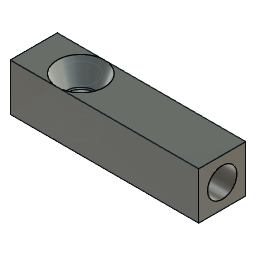
support_tige_metal (Autodesk Fusion 360 design; units mm, degrees)
Autodesk Fusion 360 part; units mm, degrees
sketch "Esquisse1" plane through (0, 0, 0) normal (0, 0, 1) x (1, 0, 0)
  line L0 (0, 0) -> (40, 0)
  line L1 (40, 0) -> (40, -10)
  line L2 (40, -10) -> (0, -10)
  line L3 (0, -10) -> (0, 0)
  circle A0 centre (10, -5) radius 3.25
  dimension "d1" = 6.5
  constraint horizontal L0
  constraint vertical L1
  constraint horizontal L2
  constraint vertical L3
  constraint coincident L0.start L3.end
  measures "d1" diameter of A0
extrude "Extrusion1" add sketch "Esquisse1" along normal blind 10
sketch "Esquisse2" plane through (40, 0, 0) normal (1, 0, 0) x (0, 1, 0)
  line L0 (-10, 0) -> (0, 0)
  line L1 (0, 0) -> (0, 10)
  line L2 (0, 10) -> (-10, 10)
  line L3 (-10, 10) -> (-10, 0)
  circle A0 centre (-5, 5) radius 3.1
  dimension "d4" = 6.2
  measures "d4" diameter of A0
extrude "Extrusion2" cut sketch "Esquisse2" against normal blind 20 contours A0
sketch "Esquisse3" plane through (0, 0, 10) normal (0, 0, 1) x (-1, 0, 0)
  circle A0 centre (-10, 5) radius 3.25
  line L0 (0, 10) -> (-40, 10)
  line L1 (-40, 10) -> (-40, 0)
  line L2 (-40, 0) -> (0, 0)
  line L3 (0, 0) -> (0, 10)
sketch "Esquisse4" plane through (0, 0, 0) normal (0, 0, -1) x (1, 0, 0)
  circle A0 centre (10, 5) radius 3.25
  line L0 (40, 10) -> (0, 10)
  line L1 (0, 10) -> (0, 0)
  line L2 (0, 0) -> (40, 0)
  line L3 (40, 0) -> (40, 10)
sketch "Esquisse5" plane through (0, 0, 10) normal (0, 0, 1) x (-1, 0, 0)
  circle A0 centre (-10, 5) radius 3.25
  dimension "d7" = 6.5
  measures "d7" diameter of A0
hole "Perçage1" at (10, -5, 10) direction (0, 0, -1) diameter 6.5 depth 73.51 tip angle 118 countersink diameter 10 countersink angle 40
sketch "Esquisse6" plane through (0, 0, 0) normal (0, 0, -1) x (1, 0, 0)
  circle A0 centre (10, 5) radius 3.25
  dimension "d13" = 6.5
  measures "d13" diameter of A0
hole "Perçage2" at (10, -5, 0) direction (0, 0, 1) diameter 6.5 depth 73.51 tip angle 118 countersink diameter 10 countersink angle 40
